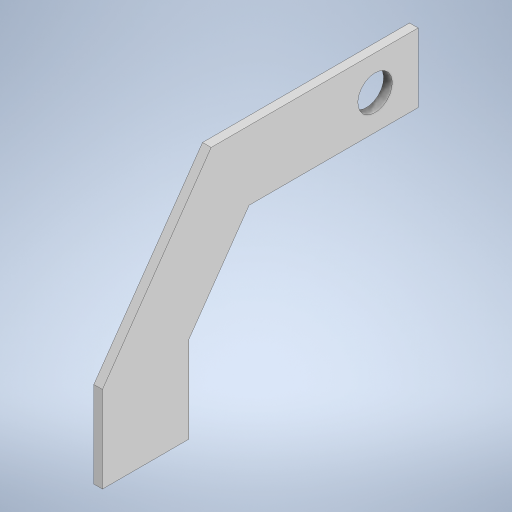
# Autodesk Inventor part: Pieza19
Saved by Autodesk Inventor 2023 (Build 270158000, 158)
## iProperties
Created: 2023-06-06
Part Number: Pieza19
Material: Genérico
Document SubType Name: Modeling
Designer: sergi
Density: 1 g/cm^3
Appearance: Valor por defecto
Author: sergi
Autodesk Inventor part; units mm, degrees
ref_plane "YZ Plane" through (0, 0, 0) normal (1, 0, 0) x (0, 1, 0)
ref_plane "XZ Plane" through (0, 0, 0) normal (0, 1, 0) x (-1, 0, 0)
ref_plane "XY Plane" through (0, 0, 0) normal (0, 0, 1) x (1, 0, 0)
sketch "Boceto1" plane through (0, 0, 0) normal (1, 0, 0) x (0, 1, 0)
  line L0 (0, 0) -> (50, 0)
  line L1 (50, 0) -> (50, -50)
  line L2 (50, -50) -> (0, -50)
  line L3 (0, -50) -> (0, 0)
  line L4 (50, 0) -> (140, -63.0187)
  line L5 (140, -63.0187) -> (140, -183.0187)
  line L6 (140, -183.0187) -> (100, -183.0187)
  line L7 (100, -183.0187) -> (100, -85.0104)
  line L8 (100, -85.0104) -> (50, -50)
  circle A0 centre (120, -158.0187) radius 10
  point P0 (120, -183.0187)
  dimension "d0" = 50
  dimension "d1" = 50
  dimension "d2" = 120
  dimension "d3" = 40
  dimension "d4" = 55
  dimension "d5" = 20
  dimension "d6" = 25
  dimension "d9" = 50
  constraints: 18 end point, 3 parallel, 3 perpendicular, 1 centre point, 1 horizontal, 1 midpoint, 1 vertical, 1 vertical alignment
  measures "d0" distance of L1.end L2.end
  measures "d1" distance of L0.end L1.end
  measures "d2" distance of L4.end L5.end
  measures "d3" distance of L5.end L6.end
  measures "d4" angle of L1 L8
  measures "d5" diameter of A0
  measures "d6" distance from line of L6 A0.centre
  measures "d9" distance between parallel lines of L7 L1
extrude "Extrusión1" add sketch "Boceto1" along normal blind 5
